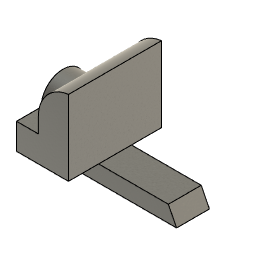
Part 11 (Autodesk Fusion 360 design; units mm, degrees)
Autodesk Fusion 360 part; units mm, degrees
sketch "Sketch1" plane through (0, 0, 0) normal (0, 1, 0) x (1, 0, 0)
  line L0 (22, 19) -> (-16, 19)
  line L1 (-16, 19) -> (-16, 0)
  line L2 (-16, 0) -> (0, 0)
  line L3 (0, 0) -> (0, -11.1807)
  arc A0 (0, -11.1807) -> (22, -36) centre (25, -11.1807) ccw
  line L4 (22, -36) -> (22, 19)
  dimension "d1" = 55
  dimension "d2" = 38
  dimension "d3" = 25
  dimension "d4" = 16
  dimension "d5" = 19
  constraint horizontal L0
  constraint perpendicular L0 L1
  constraint perpendicular L1 L2
  constraint perpendicular L2 L3
  constraint tangent L3 A0
  constraint perpendicular L0 L4
  constraint coincident L2.end L3.start
  measures "d1" distance of L0 A0.end
  measures "d2" distance of L0.start L0.end
  measures "d3" radius of A0
  measures "d4" distance of L1.end L2.end
  measures "d5" distance of L0.end L1.end
extrude "Extrude1" add sketch "Sketch1" along normal blind 34 and the other way blind 34
sketch "Sketch2" plane through (-16, 0, 0) normal (-1, 0, 0) x (0, -1, 0)
  line L0 (34, 0) -> (-34, 0)
  line L1 (-34, 0) -> (-34, -19)
  line L2 (-34, -19) -> (34, -19)
  line L3 (34, -19) -> (34, 0)
  line L4 (-12, -19) -> (12, -19)
  line L5 (12, -19) -> (12, -31)
  line L6 (12, -31) -> (-12, -31)
  line L7 (-12, -31) -> (-12, -19)
  dimension "d10" = 12
  dimension "d11" = 24
  dimension "d12" = 22
  constraint horizontal L4
  constraint vertical L5
  constraint horizontal L6
  constraint vertical L7
  constraint coincident L2 L4.start
  measures "d10" distance of L4.end L5.end
  measures "d11" distance of L5.end L6.end
  measures "d12" distance of L2.end L5
extrude "Extrude2" add sketch "Sketch2" against normal blind 95 contours L2 L4 L5 L6 L7
chamfer "Chamfer1" distance 12 distance2 6 1 edges at (79, 0, -19) measured on face at (79, 4, -23)
sketch "Sketch3" plane through (-16, 0, 0) normal (-1, 0, 0) x (0, -1, 0)
  line L0 (34, 0) -> (-34, 0)
  line L1 (-34, 0) -> (-34, -19)
  line L2 (-34, -19) -> (-12, -19)
  line L3 (-12, -19) -> (-12, -31)
  line L4 (-12, -31) -> (12, -31)
  line L5 (12, -31) -> (12, -19)
  line L6 (12, -19) -> (34, -19)
  line L7 (34, -19) -> (34, 0)
  arc A0 (16, 0) -> (-16, 0) centre (0, 0) ccw
  dimension "d17" = 32
  constraint coincident A0.centre origin
  constraint coincident L0 A0.end
  constraint coincident L0 A0.start
  measures "d17" diameter of A0
extrude "Extrude3" add sketch "Sketch3" along normal up to surface contours L0 A0 end surface at (1.4183, 11.3333, 19.4813)
sketch "Sketch4" plane through (-16, 0, 0) normal (-1, 0, 0) x (0, -1, 0)
  line L0 (34, 0) -> (16, 0)
  arc A0 (16, 0) -> (-16, 0) centre (0, 0) ccw
  line L1 (-16, 0) -> (-34, 0)
  line L2 (-34, 0) -> (-34, -19)
  line L3 (-34, -19) -> (-12, -19)
  line L4 (-12, -19) -> (-12, -31)
  line L5 (-12, -31) -> (12, -31)
  line L6 (12, -31) -> (12, -19)
  line L7 (12, -19) -> (34, -19)
  line L8 (34, -19) -> (34, 0)
  circle A1 centre (0, 0) radius 6
  dimension "d21" = 12
  constraint coincident A0.centre A1.centre
  measures "d21" diameter of A1
extrude "Extrude4" cut sketch "Sketch4" against normal blind 16 contours A1
